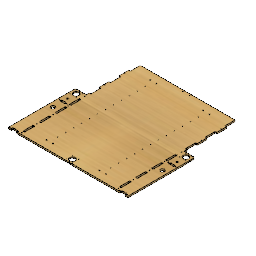
Bottom-plate-IIIS-rev1_8mm v1 (Autodesk Fusion 360 design; units mm, degrees)
Autodesk Fusion 360 part; units mm, degrees
(part 1 of 2)
sketch "Basic shape" plane through (0, 0, 0) normal (0, 1, 0) x (1, 0, 0)
  line L0 (-300, 300) -> (300, 300)
  line L1 (300, 300) -> (300, -300)
  line L2 (300, -300) -> (-300, -300)
  line L3 (-300, -300) -> (-300, 300)
  line L4 (-300, 300) -> (-246, 300)
  line L5 (-246, 300) -> (-246, 36.5)
  line L6 (-246, 36.5) -> (-300, 36.5)
  line L7 (-300, 36.5) -> (-300, 300)
  line L8 (300, 300) -> (246, 300)
  line L9 (246, 300) -> (246, 36.5)
  line L10 (246, 36.5) -> (300, 36.5)
  line L11 (300, 36.5) -> (300, 300)
  dimension "d1" = 600
  dimension "d2" = 600
  dimension "d3" = 263.5
  dimension "d4" = 54
  measures "d100" distance of origin
  measures "d166" distance of origin
extrude "Extrude1" add sketch "Basic shape" along normal blind 8 contours L0 L1 L2 L3 L5 L6 L9 L10
sketch "XZ1 plane projected" plane through (0, 8, 0) normal (0, 1, 0) x (-1, 0, 0)
  line L0 (246, -300) -> (246, -36.5)
  line L1 (246, -36.5) -> (300, -36.5)
  line L2 (300, -36.5) -> (300, 300)
  line L3 (300, 300) -> (-300, 300)
  line L4 (-300, 300) -> (-300, -36.5)
  line L5 (-300, -36.5) -> (-246, -36.5)
  line L6 (-246, -36.5) -> (-246, -300)
  line L7 (-246, -300) -> (246, -300)
  line L8 (300, 48.5) -> (-300, 48.5) construction
  line L9 (-300, 48.5) -> (-300, 56.5) construction
  line L10 (-300, 56.5) -> (300, 56.5) construction
  line L11 (300, 56.5) -> (300, 48.5) construction
  dimension "d29" = 48.5
  dimension "d30" = 8
sketch "XZ1 joints" plane through (0, 8, 0) normal (0, 1, 0) x (-1, 0, 0)
  line L0 (300, 48.5) -> (285.5, 48.5)
  line L1 (285.5, 48.5) -> (285.5, 56.5)
  line L2 (285.5, 56.5) -> (300, 56.5)
  line L3 (300, 56.5) -> (300, 48.5)
  line L4 (-300, 56.5) -> (300, 56.5)
  line L5 (260.5, 48.5) -> (246, 48.5)
  line L6 (246, 48.5) -> (246, 56.5)
  line L7 (246, 56.5) -> (260.5, 56.5)
  line L8 (260.5, 56.5) -> (260.5, 48.5)
  line L9 (300, 48.5) -> (-300, 48.5)
  dimension "d31" = 14.5
  dimension "d32" = 25
  dimension "d33" = 14.5
  measures "d32" distance of L1 L8
sketch "XZ1 joints holes" plane through (0, 8, 0) normal (0, 1, 0) x (-1, 0, 0)
  circle A0 centre (254.5, 52.5) radius 2
  circle A1 centre (291.5, 52.5) radius 2
  line L0 (246, -300) -> (246, -36.5)
  line L1 (246, -36.5) -> (300, -36.5)
  line L2 (300, -36.5) -> (300, 300)
  line L3 (300, 300) -> (-300, 300)
  line L4 (-300, 300) -> (-300, -36.5)
  line L5 (-300, -36.5) -> (-246, -36.5)
  line L6 (-246, -36.5) -> (-246, -300)
  line L7 (-246, -300) -> (246, -300)
  line L8 (300, 48.5) -> (285.5, 48.5)
  line L9 (260.5, 48.5) -> (246, 48.5)
  dimension "d34" = 4
  dimension "d64" = 4
  dimension "d71" = 4
  dimension "d72" = 4
  dimension "d1200" = 6
  dimension "d1201" = 6
  measures "d34" diameter of A0
  measures "d64" diameter of A1
extrude "Extrude2" cut sketch "XZ1 joints" sketch "XZ1 joints holes" against normal through all contours L1 L4 L8 L9 of sketch 2 contours A0 | A1
mirror "Mirror1" about plane through (0, 0, 0) normal (1, 0, 0) of "Extrude2"
sketch "XZ2 plane projected" plane through (0, 8, 0) normal (0, 1, 0) x (-1, 0, 0)
  line L0 (-246, -300) -> (246, -300)
  line L1 (246, -300) -> (246, -36.5)
  line L2 (246, -36.5) -> (300, -36.5)
  line L3 (300, -36.5) -> (300, 300)
  line L4 (300, 300) -> (-300, 300) construction
  line L5 (300, 300) -> (-300, 300) construction
  line L6 (-300, 300) -> (-300, 292) construction
  line L7 (-300, 292) -> (300, 292) construction
  line L8 (300, 292) -> (300, 300) construction
  dimension "d53" = 8
sketch "XZ2 joints" plane through (0, 8, 0) normal (0, 1, 0) x (-1, 0, 0)
  line L0 (-246, -300) -> (246, -300)
  line L1 (246, -300) -> (246, -36.5)
  line L2 (246, -36.5) -> (300, -36.5)
  line L3 (300, -36.5) -> (300, 300)
  line L4 (300, 300) -> (-300, 300)
  line L5 (300, 292) -> (285.5, 292)
  line L6 (285.5, 292) -> (285.5, 300)
  line L7 (285.5, 300) -> (300, 300)
  line L8 (300, 300) -> (300, 292)
  line L9 (260.5, 292) -> (246, 292)
  line L10 (246, 292) -> (246, 300)
  line L11 (246, 300) -> (260.5, 300)
  line L12 (260.5, 300) -> (260.5, 292)
  line L13 (-300, 292) -> (300, 292)
  dimension "d54" = 14.5
  dimension "d55" = 14.5
  dimension "d56" = 25
sketch "XZ2 joints holes" plane through (-273.5, 8, 295) normal (0, 1, 0) x (-1, 0, 0)
  circle A0 centre (18, 1) radius 2
  circle A1 centre (-19, 1) radius 2
  line L0 (26.5, -3) -> (12, -3)
  line L1 (-13, -3) -> (-27.5, -3)
  dimension "d73" = 4
  dimension "d74" = 4
  dimension "d75" = 4
  dimension "d76" = 4
  dimension "d77" = 6
  dimension "d78" = 6
  measures "d73" diameter of A0
  measures "d74" diameter of A1
  measures "d75" distance of L0
  measures "d76" distance of L1
extrude "Extrude3" cut sketch "XZ2 joints" sketch "XZ2 joints holes" against normal through all contours L4 L6 L12 L13 of sketch 2
mirror "Mirror2" about plane through (0, 0, 0) normal (1, 0, 0) of "Extrude3"
sketch "Square projected" plane through (0, 8, 0) normal (0, 1, 0) x (-1, 0, 0)
  circle A0 centre (291.5, 296) radius 2
  circle A1 centre (254.5, 296) radius 2
  circle A2 centre (-291.5, 52.5) radius 2
  line L0 (-260.5, 48.5) -> (-285.5, 48.5)
  line L1 (-285.5, 48.5) -> (-285.5, 56.5)
  line L2 (-285.5, 56.5) -> (-260.5, 56.5)
  line L3 (-260.5, 56.5) -> (-260.5, 48.5)
  circle A3 centre (-254.5, 52.5) radius 2
  circle A4 centre (291.5, 52.5) radius 2
  line L4 (260.5, 56.5) -> (285.5, 56.5)
  line L5 (285.5, 56.5) -> (285.5, 48.5)
  line L6 (285.5, 48.5) -> (260.5, 48.5)
  line L7 (260.5, 48.5) -> (260.5, 56.5)
  circle A5 centre (254.5, 52.5) radius 2
  line L8 (-260.5, 300) -> (-260.5, 292)
  line L9 (-260.5, 292) -> (-285.5, 292)
  line L10 (-285.5, 292) -> (-285.5, 300)
  line L11 (-285.5, 300) -> (-300, 300)
  line L12 (-300, 300) -> (-300, -36.5)
  line L13 (-300, -36.5) -> (-246, -36.5)
  line L14 (-246, -36.5) -> (-246, -300)
  line L15 (-246, -300) -> (246, -300)
  line L16 (246, -300) -> (246, -36.5)
  line L17 (246, -36.5) -> (300, -36.5)
  line L18 (300, -36.5) -> (300, 300)
  line L19 (300, 300) -> (285.5, 300)
  line L20 (285.5, 300) -> (285.5, 292)
  line L21 (285.5, 292) -> (260.5, 292)
  line L22 (260.5, 292) -> (260.5, 300)
  line L23 (260.5, 300) -> (-260.5, 300)
  circle A6 centre (-254.5, 296) radius 2
  circle A7 centre (-291.5, 296) radius 2
  line L24 (246, 300) -> (238, 300) construction
  line L25 (238, 300) -> (238, -300) construction
  line L26 (238, -300) -> (246, -300) construction
  line L27 (246, -300) -> (246, 300) construction
  dimension "d80" = 8
sketch "SquareBack joints" plane through (0, 8, 0) normal (0, 1, 0) x (-1, 0, 0)
  line L0 (246, 68.5) -> (238, 68.5)
  line L1 (238, 68.5) -> (238, 118.5)
  line L2 (238, 118.5) -> (246, 118.5)
  line L3 (246, 118.5) -> (246, 68.5)
  line L4 (246, -300) -> (246, 300)
  line L5 (238, 300) -> (238, -300)
  line L6 (246, 149.25) -> (238, 149.25)
  line L7 (238, 149.25) -> (238, 199.25)
  line L8 (238, 199.25) -> (246, 199.25)
  line L9 (246, 199.25) -> (246, 149.25)
  line L10 (246, 230) -> (238, 230)
  line L11 (238, 230) -> (238, 280)
  line L12 (238, 280) -> (246, 280)
  line L13 (246, 280) -> (246, 230)
  line L14 (238, 199.25) -> (238, 230) construction
  line L15 (238, 230) -> (238, 199.25)
  line L16 (238, 118.5) -> (238, 149.25) construction
  dimension "d81" = 50
  dimension "d1204" = 20
  dimension "d1205" = 20
  dimension "d1918" = 30.75
extrude "Extrude4" cut sketch "SquareBack joints" against normal through all contours L0 L1 L2 L3 L4 L5 | L4 L5 L6 L7 L8 L9 | L4 L5 L10 L11 L12 L13
sketch "SquareBack joints holes" plane through (0, 8, 0) normal (0, 1, 0) x (-1, 0, 0)
  line L0 (246, 68.5) -> (238, 68.5)
  line L1 (238, 68.5) -> (238, 118.5)
  line L2 (238, 118.5) -> (246, 118.5)
  line L3 (246, 118.5) -> (246, 68.5)
  line L4 (246, 199.25) -> (246, 149.25)
  line L5 (246, 149.25) -> (238, 149.25)
  line L6 (238, 149.25) -> (238, 199.25)
  line L7 (238, 199.25) -> (246, 199.25)
  line L8 (246, 280) -> (246, 230)
  line L9 (246, 230) -> (238, 230)
  line L10 (238, 230) -> (238, 280)
  line L11 (238, 280) -> (246, 280)
  circle A0 centre (291.5, 296) radius 2
  circle A1 centre (254.5, 296) radius 2
  circle A2 centre (-291.5, 52.5) radius 2
  line L12 (-260.5, 48.5) -> (-285.5, 48.5)
  line L13 (-285.5, 48.5) -> (-285.5, 56.5)
  line L14 (-285.5, 56.5) -> (-260.5, 56.5)
  line L15 (-260.5, 56.5) -> (-260.5, 48.5)
  circle A3 centre (-254.5, 52.5) radius 2
  circle A4 centre (291.5, 52.5) radius 2
  line L16 (260.5, 56.5) -> (285.5, 56.5)
  line L17 (285.5, 56.5) -> (285.5, 48.5)
  line L18 (285.5, 48.5) -> (260.5, 48.5)
  line L19 (260.5, 48.5) -> (260.5, 56.5)
  circle A5 centre (254.5, 52.5) radius 2
  line L20 (-260.5, 300) -> (-260.5, 292)
  line L21 (-260.5, 292) -> (-285.5, 292)
  line L22 (-285.5, 292) -> (-285.5, 300)
  line L23 (-285.5, 300) -> (-300, 300)
  line L24 (-300, 300) -> (-300, -36.5)
  line L25 (-300, -36.5) -> (-246, -36.5)
  line L26 (-246, -36.5) -> (-246, -300)
  line L27 (-246, -300) -> (246, -300)
  line L28 (246, -300) -> (246, -36.5)
  line L29 (246, -36.5) -> (300, -36.5)
  line L30 (300, -36.5) -> (300, 300)
  line L31 (300, 300) -> (285.5, 300)
  line L32 (285.5, 300) -> (285.5, 292)
  line L33 (285.5, 292) -> (260.5, 292)
  line L34 (260.5, 292) -> (260.5, 300)
  line L35 (260.5, 300) -> (-260.5, 300)
  circle A6 centre (-254.5, 296) radius 2
  circle A7 centre (-291.5, 296) radius 2
  circle A8 centre (242, 58.5) radius 2
  circle A9 centre (242, 133.875) radius 2
  circle A10 centre (242, 290) radius 2
  circle A11 centre (242, 214.625) radius 2
  line L36 (246, 68.5) -> (238, 68.5)
  line L37 (238, 118.5) -> (238, 149.25) construction
  line L38 (238, 199.25) -> (238, 230) construction
  dimension "d86" = 4
  dimension "d87" = 4
  dimension "d88" = 4
  dimension "d89" = 4
  dimension "d727" = 10
  dimension "d728" = 10
  dimension "d1206" = 14.625
  dimension "d1207" = 14.625
  dimension "d1208" = 14.625
  dimension "d1209" = 14.625
  measures "d86" diameter of A10
  measures "d87" diameter of A11
  measures "d88" diameter of A9
  measures "d89" diameter of A8
extrude "Extrude5" cut sketch "SquareBack joints holes" against normal through all contours A8 | A9 | A10 | A11
mirror "Mirror3" about plane through (0, 0, 0) normal (1, 0, 0) of "Extrude4", "Extrude5"
sketch "SquareFront joints" plane through (0, 0, 0) normal (0, 1, 0) x (1, 0, 0)
  line L0 (-238, 300) -> (-246, 300)
  line L1 (-246, 300) -> (-246, 200.5)
  line L2 (-246, 200.5) -> (-238, 200.5)
  line L3 (-238, 200.5) -> (-238, 300)
  line L4 (-246, 300) -> (-246, 36.5)
  line L5 (-246, 300) -> (-246, -300)
  line L6 (-238, 250) -> (-246, 250)
  line L7 (-246, 250) -> (-246, 150.5)
  line L8 (-246, 150.5) -> (-238, 150.5)
  line L9 (-238, 150.5) -> (-238, 250)
  line L10 (-238, -300) -> (-238, 300)
  line L11 (-238, 101) -> (-246, 101)
  line L12 (-246, 101) -> (-246, 51)
  line L13 (-246, 51) -> (-238, 51)
  line L14 (-238, 51) -> (-238, 101)
  line L15 (-238, 1.5) -> (-246, 1.5)
  line L16 (-246, 1.5) -> (-246, -48.5)
  line L17 (-246, -48.5) -> (-238, -48.5)
  line L18 (-238, -48.5) -> (-238, 1.5)
  line L19 (-238, 200.5) -> (-238, 250) construction
  line L20 (-238, 150.5) -> (-238, 101) construction
  line L21 (-238, 51) -> (-238, 1.5) construction
  dimension "d94" = 50
  dimension "d98" = 50
  dimension "d99" = 50
  dimension "d100" = 50
  measures "d98" distance of L2 L8
  measures "d99" distance of L11 L13
  measures "d100" distance of L15 L17
extrude "Extrude6" cut sketch "SquareFront joints" along normal through all contours L0 L1 L3 L4 L5 L6 L10 | L2 L4 L5 L7 L8 L9 L10 | L4 L5 L10 L11 L12 L13 L14 | L5 L10 L15 L16 L17 L18
sketch "SquareFront joints holes" plane through (0, 0, 0) normal (0, -1, 0) x (1, 0, 0)
  circle A0 centre (-254.5, 52.5) radius 2
  line L0 (-285.5, 56.5) -> (-260.5, 56.5)
  line L1 (-260.5, 56.5) -> (-260.5, 48.5)
  line L2 (-260.5, 48.5) -> (-285.5, 48.5)
  line L3 (-285.5, 48.5) -> (-285.5, 56.5)
  circle A1 centre (-291.5, 52.5) radius 2
  circle A2 centre (254.5, 52.5) radius 2
  line L4 (285.5, 48.5) -> (260.5, 48.5)
  line L5 (260.5, 48.5) -> (260.5, 56.5)
  line L6 (260.5, 56.5) -> (285.5, 56.5)
  line L7 (285.5, 56.5) -> (285.5, 48.5)
  circle A3 centre (291.5, 52.5) radius 2
  circle A4 centre (-254.5, 296) radius 2
  circle A5 centre (-291.5, 296) radius 2
  circle A6 centre (254.5, 296) radius 2
  circle A7 centre (291.5, 296) radius 2
  line L8 (-246, 230) -> (-246, 280)
  line L9 (-246, 280) -> (-238, 280)
  line L10 (-238, 280) -> (-238, 230)
  line L11 (-238, 230) -> (-246, 230)
  line L12 (-246, 149.25) -> (-246, 199.25)
  line L13 (-246, 199.25) -> (-238, 199.25)
  line L14 (-238, 199.25) -> (-238, 149.25)
  line L15 (-238, 149.25) -> (-246, 149.25)
  line L16 (-238, 68.5) -> (-246, 68.5)
  line L17 (-246, 68.5) -> (-246, 118.5)
  line L18 (-246, 118.5) -> (-238, 118.5)
  line L19 (-238, 118.5) -> (-238, 68.5)
  circle A8 centre (-242, 290) radius 2
  circle A9 centre (-242, 58.5) radius 2
  circle A10 centre (-242, 214.625) radius 2
  circle A11 centre (-242, 133.875) radius 2
  line L20 (238, 230) -> (238, 280)
  line L21 (238, 280) -> (246, 280)
  line L22 (246, 280) -> (246, 230)
  line L23 (246, 230) -> (238, 230)
  line L24 (238, 149.25) -> (238, 199.25)
  line L25 (238, 199.25) -> (246, 199.25)
  line L26 (246, 199.25) -> (246, 149.25)
  line L27 (246, 149.25) -> (238, 149.25)
  line L28 (238, 118.5) -> (246, 118.5)
  line L29 (246, 118.5) -> (246, 68.5)
  line L30 (246, 68.5) -> (238, 68.5)
  line L31 (238, 68.5) -> (238, 118.5)
  circle A12 centre (242, 290) radius 2
  circle A13 centre (242, 58.5) radius 2
  circle A14 centre (242, 214.625) radius 2
  circle A15 centre (242, 133.875) radius 2
  line L32 (-246, 48.5) -> (-238, 48.5)
  line L33 (-238, 48.5) -> (-238, -1.5)
  line L34 (-238, -1.5) -> (-246, -1.5)
  line L35 (-246, -1.5) -> (-246, 48.5)
  line L36 (246, -300) -> (246, -36.5)
  line L37 (246, -36.5) -> (300, -36.5)
  line L38 (300, -36.5) -> (300, 300)
  line L39 (300, 300) -> (285.5, 300)
  line L40 (285.5, 300) -> (285.5, 292)
  line L41 (285.5, 292) -> (260.5, 292)
  line L42 (260.5, 292) -> (260.5, 300)
  line L43 (260.5, 300) -> (-260.5, 300)
  line L44 (-260.5, 300) -> (-260.5, 292)
  line L45 (-260.5, 292) -> (-285.5, 292)
  line L46 (-285.5, 292) -> (-285.5, 300)
  line L47 (-285.5, 300) -> (-300, 300)
  line L48 (-300, 300) -> (-300, -36.5)
  line L49 (-300, -36.5) -> (-246, -36.5)
  line L50 (-246, -36.5) -> (-246, -51)
  line L51 (-246, -51) -> (-238, -51)
  line L52 (-238, -51) -> (-238, -101)
  line L53 (-238, -101) -> (-246, -101)
  line L54 (-246, -101) -> (-246, -150.5)
  line L55 (-246, -150.5) -> (-238, -150.5)
  line L56 (-238, -150.5) -> (-238, -200.5)
  line L57 (-238, -200.5) -> (-246, -200.5)
  line L58 (-246, -200.5) -> (-246, -250)
  line L59 (-246, -250) -> (-238, -250)
  line L60 (-238, -250) -> (-238, -300)
  line L61 (-238, -300) -> (246, -300)
  circle A16 centre (-242, -225.25) radius 2
  circle A17 centre (-242, -125.75) radius 2
  circle A18 centre (-242, -26.25) radius 2
  line L62 (-238, -250) -> (-238, -200.5) construction
  line L63 (-238, -150.5) -> (-238, -101) construction
  line L64 (-238, -51) -> (-238, -1.5) construction
  dimension "d105" = 4
  dimension "d106" = 4
  dimension "d107" = 4
  dimension "d108" = 4
  dimension "d109" = 4
  dimension "d110" = 4
  measures "d108" diameter of A18
  measures "d109" diameter of A17
  measures "d110" diameter of A16
extrude "Extrude7" cut sketch "SquareFront joints holes" against normal through all contours A16 | A17 | A18
mirror "Mirror5" about plane through (0, 0, 0) normal (1, 0, 0) of "Extrude6", "Extrude7"
sketch "SK8" plane through (0, 8, 0) normal (0, 1, 0) x (-1, 0, 0)
  circle A0 centre (-242, -225.25) radius 2
  circle A1 centre (-242, -125.75) radius 2
  circle A2 centre (-242, -26.25) radius 2
  circle A3 centre (242, -225.25) radius 2
  circle A4 centre (242, -125.75) radius 2
  circle A5 centre (242, -26.25) radius 2
  circle A6 centre (-242, 133.875) radius 2
  circle A7 centre (-242, 214.625) radius 2
  circle A8 centre (-242, 58.5) radius 2
  circle A9 centre (-242, 290) radius 2
  line L0 (-246, 118.5) -> (-238, 118.5)
  line L1 (-238, 118.5) -> (-238, 68.5)
  line L2 (-238, 68.5) -> (-246, 68.5)
  line L3 (-246, 68.5) -> (-246, 118.5)
  line L4 (-238, 199.25) -> (-238, 149.25)
  line L5 (-238, 149.25) -> (-246, 149.25)
  line L6 (-246, 149.25) -> (-246, 199.25)
  line L7 (-246, 199.25) -> (-238, 199.25)
  line L8 (-238, 280) -> (-238, 230)
  line L9 (-238, 230) -> (-246, 230)
  line L10 (-246, 230) -> (-246, 280)
  line L11 (-246, 280) -> (-238, 280)
  circle A10 centre (242, 133.875) radius 2
  circle A11 centre (242, 214.625) radius 2
  circle A12 centre (242, 58.5) radius 2
  circle A13 centre (242, 290) radius 2
  line L12 (246, 68.5) -> (238, 68.5)
  line L13 (238, 68.5) -> (238, 118.5)
  line L14 (238, 118.5) -> (246, 118.5)
  line L15 (246, 118.5) -> (246, 68.5)
  line L16 (246, 199.25) -> (246, 149.25)
  line L17 (246, 149.25) -> (238, 149.25)
  line L18 (238, 149.25) -> (238, 199.25)
  line L19 (238, 199.25) -> (246, 199.25)
  line L20 (246, 280) -> (246, 230)
  line L21 (246, 230) -> (238, 230)
  line L22 (238, 230) -> (238, 280)
  line L23 (238, 280) -> (246, 280)
  circle A14 centre (291.5, 296) radius 2
  circle A15 centre (254.5, 296) radius 2
  circle A16 centre (-291.5, 52.5) radius 2
  line L24 (-260.5, 48.5) -> (-285.5, 48.5)
  line L25 (-285.5, 48.5) -> (-285.5, 56.5)
  line L26 (-285.5, 56.5) -> (-260.5, 56.5)
  line L27 (-260.5, 56.5) -> (-260.5, 48.5)
  circle A17 centre (-254.5, 52.5) radius 2
  circle A18 centre (291.5, 52.5) radius 2
  line L28 (260.5, 56.5) -> (285.5, 56.5)
  line L29 (285.5, 56.5) -> (285.5, 48.5)
  line L30 (285.5, 48.5) -> (260.5, 48.5)
  line L31 (260.5, 48.5) -> (260.5, 56.5)
  circle A19 centre (254.5, 52.5) radius 2
  line L32 (-260.5, 300) -> (-260.5, 292)
  line L33 (-260.5, 292) -> (-285.5, 292)
  line L34 (-285.5, 292) -> (-285.5, 300)
  line L35 (-285.5, 300) -> (-300, 300)
  line L36 (-300, 300) -> (-300, -36.5)
  line L37 (-300, -36.5) -> (-246, -36.5)
  line L38 (-246, -36.5) -> (-246, -51)
  line L39 (-238, -300) -> (238, -300)
  line L40 (246, -250) -> (246, -200.5)
  line L41 (246, -36.5) -> (300, -36.5)
  line L42 (300, -36.5) -> (300, 300)
  line L43 (300, 300) -> (285.5, 300)
  line L44 (285.5, 300) -> (285.5, 292)
  line L45 (285.5, 292) -> (260.5, 292)
  line L46 (260.5, 292) -> (260.5, 300)
  line L47 (260.5, 300) -> (-260.5, 300)
  circle A20 centre (-254.5, 296) radius 2
  circle A21 centre (-291.5, 296) radius 2
  line L48 (-149, -260) -> (-117, -260) construction
  circle A22 centre (-149, -260) radius 2.5
  circle A23 centre (-117, -260) radius 2.5
  line L49 (246, -1.5) -> (238, -1.5)
  line L50 (238, -1.5) -> (238, 48.5)
  line L51 (238, 48.5) -> (246, 48.5)
  line L52 (246, 48.5) -> (246, -1.5)
  line L53 (-246, 48.5) -> (-238, 48.5)
  line L54 (-238, 48.5) -> (-238, -1.5)
  line L55 (-238, -1.5) -> (-246, -1.5)
  line L56 (-246, -1.5) -> (-246, 48.5)
  line L57 (-246, -250) -> (-238, -250)
  line L58 (-238, -250) -> (-238, -300)
  line L59 (238, -300) -> (238, -250)
  line L60 (238, -250) -> (246, -250)
  line L61 (246, -200.5) -> (238, -200.5)
  line L62 (238, -200.5) -> (238, -150.5)
  line L63 (238, -150.5) -> (246, -150.5)
  line L64 (246, -150.5) -> (246, -101)
  line L65 (246, -101) -> (238, -101)
  line L66 (238, -101) -> (238, -51)
  line L67 (238, -51) -> (246, -51)
  line L68 (246, -51) -> (246, -36.5)
  line L69 (-246, -51) -> (-238, -51)
  line L70 (-238, -51) -> (-238, -101)
  line L71 (-238, -101) -> (-246, -101)
  line L72 (-246, -101) -> (-246, -150.5)
  line L73 (-246, -150.5) -> (-238, -150.5)
  line L74 (-238, -150.5) -> (-238, -200.5)
  line L75 (-238, -200.5) -> (-246, -200.5)
  line L76 (-246, -200.5) -> (-246, -250)
  dimension "d113" = 5
  dimension "d114" = 5
  dimension "d115" = 32
  dimension "d116" = 40
  dimension "d117" = 133
  dimension "d130" = 200
  measures "d113" diameter of A22
  measures "d114" diameter of A23
  measures "d116" distance of L39 L48
extrude "Extrude8" cut sketch "SK8" against normal through all contours A22 | A23
mirror "Mirror6" about plane through (0, 0, 0) normal (1, 0, 0) of "Extrude8"
mirror "Mirror7" about plane through (0, 0, 0) normal (0, 0, 1) of "Extrude8"
mirror "Mirror8" about plane through (0, 0, 0) normal (0, 0, 1) of "Mirror6"
sketch "Linear rail" plane through (0, 8, 0) normal (0, 1, 0) x (-1, 0, 0)
  circle A0 centre (149, 260) radius 2.5
  circle A1 centre (117, 260) radius 2.5
  circle A2 centre (-149, 260) radius 2.5
  circle A3 centre (-117, 260) radius 2.5
  circle A4 centre (149, -260) radius 2.5
  circle A5 centre (117, -260) radius 2.5
  circle A6 centre (-149, -260) radius 2.5
  circle A7 centre (-117, -260) radius 2.5
  circle A8 centre (-242, -225.25) radius 2
  circle A9 centre (-242, -125.75) radius 2
  circle A10 centre (-242, -26.25) radius 2
  circle A11 centre (242, -225.25) radius 2
  circle A12 centre (242, -125.75) radius 2
  circle A13 centre (242, -26.25) radius 2
  circle A14 centre (-242, 133.875) radius 2
  circle A15 centre (-242, 214.625) radius 2
  circle A16 centre (-242, 58.5) radius 2
  circle A17 centre (-242, 290) radius 2
  line L0 (-246, 118.5) -> (-238, 118.5)
  line L1 (-238, 118.5) -> (-238, 68.5)
  line L2 (-238, 68.5) -> (-246, 68.5)
  line L3 (-246, 68.5) -> (-246, 118.5)
  line L4 (-238, 199.25) -> (-238, 149.25)
  line L5 (-238, 149.25) -> (-246, 149.25)
  line L6 (-246, 149.25) -> (-246, 199.25)
  line L7 (-246, 199.25) -> (-238, 199.25)
  line L8 (-238, 280) -> (-238, 230)
  line L9 (-238, 230) -> (-246, 230)
  line L10 (-246, 230) -> (-246, 280)
  line L11 (-246, 280) -> (-238, 280)
  circle A18 centre (242, 133.875) radius 2
  circle A19 centre (242, 214.625) radius 2
  circle A20 centre (242, 58.5) radius 2
  circle A21 centre (242, 290) radius 2
  line L12 (246, 68.5) -> (238, 68.5)
  line L13 (238, 68.5) -> (238, 118.5)
  line L14 (238, 118.5) -> (246, 118.5)
  line L15 (246, 118.5) -> (246, 68.5)
  line L16 (246, 199.25) -> (246, 149.25)
  line L17 (246, 149.25) -> (238, 149.25)
  line L18 (238, 149.25) -> (238, 199.25)
  line L19 (238, 199.25) -> (246, 199.25)
  line L20 (246, 280) -> (246, 230)
  line L21 (246, 230) -> (238, 230)
  line L22 (238, 230) -> (238, 280)
  line L23 (238, 280) -> (246, 280)
  circle A22 centre (291.5, 296) radius 2
  circle A23 centre (254.5, 296) radius 2
  circle A24 centre (-291.5, 52.5) radius 2
  line L24 (-260.5, 48.5) -> (-285.5, 48.5)
  line L25 (-285.5, 48.5) -> (-285.5, 56.5)
  line L26 (-285.5, 56.5) -> (-260.5, 56.5)
  line L27 (-260.5, 56.5) -> (-260.5, 48.5)
  circle A25 centre (-254.5, 52.5) radius 2
  circle A26 centre (291.5, 52.5) radius 2
  line L28 (260.5, 56.5) -> (285.5, 56.5)
  line L29 (285.5, 56.5) -> (285.5, 48.5)
  line L30 (285.5, 48.5) -> (260.5, 48.5)
  line L31 (260.5, 48.5) -> (260.5, 56.5)
  circle A27 centre (254.5, 52.5) radius 2
  line L32 (-260.5, 300) -> (-260.5, 292)
  line L33 (-260.5, 292) -> (-285.5, 292)
  line L34 (-285.5, 292) -> (-285.5, 300)
  line L35 (-285.5, 300) -> (-300, 300)
  line L36 (-300, 300) -> (-300, -36.5)
  line L37 (-300, -36.5) -> (-246, -36.5)
  line L38 (-246, -36.5) -> (-246, -51)
  line L39 (-238, -300) -> (238, -300)
  line L40 (246, -250) -> (246, -200.5)
  line L41 (246, -36.5) -> (300, -36.5)
  line L42 (300, -36.5) -> (300, 300)
  line L43 (300, 300) -> (285.5, 300)
  line L44 (285.5, 300) -> (285.5, 292)
  line L45 (285.5, 292) -> (260.5, 292)
  line L46 (260.5, 292) -> (260.5, 300)
  line L47 (260.5, 300) -> (-260.5, 300)
  circle A28 centre (-254.5, 296) radius 2
  circle A29 centre (-291.5, 296) radius 2
  circle A30 centre (-133, -220) radius 1.5
  line L48 (246, -1.5) -> (238, -1.5)
  line L49 (238, -1.5) -> (238, 48.5)
  line L50 (238, 48.5) -> (246, 48.5)
  line L51 (246, 48.5) -> (246, -1.5)
  line L52 (-246, 48.5) -> (-238, 48.5)
  line L53 (-238, 48.5) -> (-238, -1.5)
  line L54 (-238, -1.5) -> (-246, -1.5)
  line L55 (-246, -1.5) -> (-246, 48.5)
  line L56 (-246, -250) -> (-238, -250)
  line L57 (-238, -250) -> (-238, -300)
  line L58 (238, -300) -> (238, -250)
  line L59 (238, -250) -> (246, -250)
  line L60 (246, -200.5) -> (238, -200.5)
  line L61 (238, -200.5) -> (238, -150.5)
  line L62 (238, -150.5) -> (246, -150.5)
  line L63 (246, -150.5) -> (246, -101)
  line L64 (246, -101) -> (238, -101)
  line L65 (238, -101) -> (238, -51)
  line L66 (238, -51) -> (246, -51)
  line L67 (246, -51) -> (246, -36.5)
  line L68 (-246, -51) -> (-238, -51)
  line L69 (-238, -51) -> (-238, -101)
  line L70 (-238, -101) -> (-246, -101)
  line L71 (-246, -101) -> (-246, -150.5)
  line L72 (-246, -150.5) -> (-238, -150.5)
  line L73 (-238, -150.5) -> (-238, -200.5)
  line L74 (-238, -200.5) -> (-246, -200.5)
  line L75 (-246, -200.5) -> (-246, -250)
  dimension "d123" = 133
  dimension "d124" = 3
  dimension "d131" = 80
  measures "d124" diameter of A30
extrude "Extrude9" cut sketch "Linear rail" against normal through all contours A30
pattern_linear "R-Pattern1" count 12 spacing 40 along (0, 0, 1) of "Extrude9"
mirror "Mirror9" about plane through (0, 0, 0) normal (1, 0, 0) of "Extrude9", "R-Pattern1"
sketch "Y cable stretcher" plane through (0, 8, 0) normal (0, 1, 0) x (-1, 0, 0)
  circle A0 centre (133, 100) radius 1.5
  circle A1 centre (133, 60) radius 1.5
  circle A2 centre (133, 20) radius 1.5
  circle A3 centre (133, -20) radius 1.5
  circle A4 centre (133, -60) radius 1.5
  circle A5 centre (133, -100) radius 1.5
  circle A6 centre (133, -140) radius 1.5
  circle A7 centre (133, -180) radius 1.5
  circle A8 centre (133, -220) radius 1.5
  circle A9 centre (-133, 100) radius 1.5
  circle A10 centre (-133, 60) radius 1.5
  circle A11 centre (-133, 20) radius 1.5
  circle A12 centre (-133, -20) radius 1.5
  circle A13 centre (-133, -60) radius 1.5
  circle A14 centre (-133, -100) radius 1.5
  circle A15 centre (-133, -140) radius 1.5
  circle A16 centre (-133, -180) radius 1.5
  circle A17 centre (-133, -220) radius 1.5
  circle A18 centre (149, 260) radius 2.5
  circle A19 centre (117, 260) radius 2.5
  circle A20 centre (-149, 260) radius 2.5
  circle A21 centre (-117, 260) radius 2.5
  circle A22 centre (149, -260) radius 2.5
  circle A23 centre (117, -260) radius 2.5
  circle A24 centre (-149, -260) radius 2.5
  circle A25 centre (-117, -260) radius 2.5
  circle A26 centre (-242, -225.25) radius 2
  circle A27 centre (-242, -125.75) radius 2
  circle A28 centre (-242, -26.25) radius 2
  circle A29 centre (242, -225.25) radius 2
  circle A30 centre (242, -125.75) radius 2
  circle A31 centre (242, -26.25) radius 2
  circle A32 centre (-242, 133.875) radius 2
  circle A33 centre (-242, 214.625) radius 2
  circle A34 centre (-242, 58.5) radius 2
  circle A35 centre (-242, 290) radius 2
  line L0 (-246, 118.5) -> (-238, 118.5)
  line L1 (-238, 118.5) -> (-238, 68.5)
  line L2 (-238, 68.5) -> (-246, 68.5)
  line L3 (-246, 68.5) -> (-246, 118.5)
  line L4 (-238, 199.25) -> (-238, 149.25)
  line L5 (-238, 149.25) -> (-246, 149.25)
  line L6 (-246, 149.25) -> (-246, 199.25)
  line L7 (-246, 199.25) -> (-238, 199.25)
  line L8 (-238, 280) -> (-238, 230)
  line L9 (-238, 230) -> (-246, 230)
  line L10 (-246, 230) -> (-246, 280)
  line L11 (-246, 280) -> (-238, 280)
  circle A36 centre (242, 133.875) radius 2
  circle A37 centre (242, 214.625) radius 2
  circle A38 centre (242, 58.5) radius 2
  circle A39 centre (242, 290) radius 2
  line L12 (246, 68.5) -> (238, 68.5)
  line L13 (238, 68.5) -> (238, 118.5)
  line L14 (238, 118.5) -> (246, 118.5)
  line L15 (246, 118.5) -> (246, 68.5)
  line L16 (246, 199.25) -> (246, 149.25)
  line L17 (246, 149.25) -> (238, 149.25)
  line L18 (238, 149.25) -> (238, 199.25)
  line L19 (238, 199.25) -> (246, 199.25)
  line L20 (246, 280) -> (246, 230)
  line L21 (246, 230) -> (238, 230)
  line L22 (238, 230) -> (238, 280)
  line L23 (238, 280) -> (246, 280)
  circle A40 centre (291.5, 296) radius 2
  circle A41 centre (254.5, 296) radius 2
  circle A42 centre (-291.5, 52.5) radius 2
  line L24 (-260.5, 48.5) -> (-285.5, 48.5)
  line L25 (-285.5, 48.5) -> (-285.5, 56.5)
  line L26 (-285.5, 56.5) -> (-260.5, 56.5)
  line L27 (-260.5, 56.5) -> (-260.5, 48.5)
  circle A43 centre (-254.5, 52.5) radius 2
  circle A44 centre (291.5, 52.5) radius 2
  line L28 (260.5, 56.5) -> (285.5, 56.5)
  line L29 (285.5, 56.5) -> (285.5, 48.5)
  line L30 (285.5, 48.5) -> (260.5, 48.5)
  line L31 (260.5, 48.5) -> (260.5, 56.5)
  circle A45 centre (254.5, 52.5) radius 2
  line L32 (-260.5, 300) -> (-260.5, 292)
  line L33 (-260.5, 292) -> (-285.5, 292)
  line L34 (-285.5, 292) -> (-285.5, 300)
  line L35 (-285.5, 300) -> (-300, 300)
  line L36 (-300, 300) -> (-300, -36.5)
  line L37 (-300, -36.5) -> (-246, -36.5)
  line L38 (-246, -36.5) -> (-246, -51)
  line L39 (-238, -300) -> (238, -300)
  line L40 (246, -250) -> (246, -200.5)
  line L41 (246, -36.5) -> (300, -36.5)
  line L42 (300, -36.5) -> (300, 300)
  line L43 (300, 300) -> (285.5, 300)
  line L44 (285.5, 300) -> (285.5, 292)
  line L45 (285.5, 292) -> (260.5, 292)
  line L46 (260.5, 292) -> (260.5, 300)
  line L47 (260.5, 300) -> (-260.5, 300)
  circle A46 centre (-254.5, 296) radius 2
  circle A47 centre (-291.5, 296) radius 2
  circle A48 centre (133, 140) radius 1.5
  circle A49 centre (-133, 140) radius 1.5
  circle A50 centre (133, 180) radius 1.5
  circle A51 centre (-133, 180) radius 1.5
  circle A52 centre (-16, -292.5) radius 2
  circle A53 centre (133, 220) radius 1.5
  circle A54 centre (-133, 220) radius 1.5
  line L48 (246, -1.5) -> (238, -1.5)
  line L49 (238, -1.5) -> (238, 48.5)
  line L50 (238, 48.5) -> (246, 48.5)
  line L51 (246, 48.5) -> (246, -1.5)
  line L52 (-246, 48.5) -> (-238, 48.5)
  line L53 (-238, 48.5) -> (-238, -1.5)
  line L54 (-238, -1.5) -> (-246, -1.5)
  line L55 (-246, -1.5) -> (-246, 48.5)
  line L56 (-246, -250) -> (-238, -250)
  line L57 (-238, -250) -> (-238, -300)
  line L58 (238, -300) -> (238, -250)
  line L59 (238, -250) -> (246, -250)
  line L60 (246, -200.5) -> (238, -200.5)
  line L61 (238, -200.5) -> (238, -150.5)
  line L62 (238, -150.5) -> (246, -150.5)
  line L63 (246, -150.5) -> (246, -101)
  line L64 (246, -101) -> (238, -101)
  line L65 (238, -101) -> (238, -51)
  line L66 (238, -51) -> (246, -51)
  line L67 (246, -51) -> (246, -36.5)
  line L68 (-246, -51) -> (-238, -51)
  line L69 (-238, -51) -> (-238, -101)
  line L70 (-238, -101) -> (-246, -101)
  line L71 (-246, -101) -> (-246, -150.5)
  line L72 (-246, -150.5) -> (-238, -150.5)
  line L73 (-238, -150.5) -> (-238, -200.5)
  line L74 (-238, -200.5) -> (-246, -200.5)
  line L75 (-246, -200.5) -> (-246, -250)
  dimension "d134" = 7.5
  dimension "d732" = 4
  dimension "d733" = 16
  measures "d732" diameter of A52
  measures "d733" distance of origin
extrude "Extrude10" cut sketch "Y cable stretcher" against normal through all contours A52
mirror "Mirror10" about plane through (0, 0, 0) normal (1, 0, 0) of "Extrude10"
sketch "To pass cables" plane through (0, 8, 0) normal (0, 1, 0) x (-1, 0, 0)
  circle A0 centre (133, 100) radius 1.5
  circle A1 centre (133, 60) radius 1.5
  circle A2 centre (133, 20) radius 1.5
  circle A3 centre (133, -20) radius 1.5
  circle A4 centre (133, -60) radius 1.5
  circle A5 centre (133, -100) radius 1.5
  circle A6 centre (133, -140) radius 1.5
  circle A7 centre (133, -180) radius 1.5
  circle A8 centre (133, -220) radius 1.5
  circle A9 centre (-133, 100) radius 1.5
  circle A10 centre (-133, 60) radius 1.5
  circle A11 centre (-133, 20) radius 1.5
  circle A12 centre (-133, -20) radius 1.5
  circle A13 centre (-133, -60) radius 1.5
  circle A14 centre (-133, -100) radius 1.5
  circle A15 centre (-133, -140) radius 1.5
  circle A16 centre (-133, -180) radius 1.5
  circle A17 centre (-133, -220) radius 1.5
  circle A18 centre (149, 260) radius 2.5
  circle A19 centre (117, 260) radius 2.5
  circle A20 centre (-149, 260) radius 2.5
  circle A21 centre (-117, 260) radius 2.5
  circle A22 centre (149, -260) radius 2.5
  circle A23 centre (117, -260) radius 2.5
  circle A24 centre (-149, -260) radius 2.5
  circle A25 centre (-117, -260) radius 2.5
  circle A26 centre (-242, -225.25) radius 2
  circle A27 centre (-242, -125.75) radius 2
  circle A28 centre (-242, -26.25) radius 2
  circle A29 centre (242, -225.25) radius 2
  circle A30 centre (242, -125.75) radius 2
  circle A31 centre (242, -26.25) radius 2
  circle A32 centre (-242, 133.875) radius 2
  circle A33 centre (-242, 214.625) radius 2
  circle A34 centre (-242, 58.5) radius 2
  circle A35 centre (-242, 290) radius 2
  line L0 (-246, 118.5) -> (-238, 118.5)
  line L1 (-238, 118.5) -> (-238, 68.5)
  line L2 (-238, 68.5) -> (-246, 68.5)
  line L3 (-246, 68.5) -> (-246, 118.5)
  line L4 (-238, 199.25) -> (-238, 149.25)
  line L5 (-238, 149.25) -> (-246, 149.25)
  line L6 (-246, 149.25) -> (-246, 199.25)
  line L7 (-246, 199.25) -> (-238, 199.25)
  line L8 (-238, 280) -> (-238, 230)
  line L9 (-238, 230) -> (-246, 230)
  line L10 (-246, 230) -> (-246, 280)
  line L11 (-246, 280) -> (-238, 280)
  circle A36 centre (242, 133.875) radius 2
  circle A37 centre (242, 214.625) radius 2
  circle A38 centre (242, 58.5) radius 2
  circle A39 centre (242, 290) radius 2
  line L12 (246, 68.5) -> (238, 68.5)
  line L13 (238, 68.5) -> (238, 118.5)
  line L14 (238, 118.5) -> (246, 118.5)
  line L15 (246, 118.5) -> (246, 68.5)
  line L16 (246, 199.25) -> (246, 149.25)
  line L17 (246, 149.25) -> (238, 149.25)
  line L18 (238, 149.25) -> (238, 199.25)
  line L19 (238, 199.25) -> (246, 199.25)
  line L20 (246, 280) -> (246, 230)
  line L21 (246, 230) -> (238, 230)
  line L22 (238, 230) -> (238, 280)
  line L23 (238, 280) -> (246, 280)
  circle A40 centre (291.5, 296) radius 2
  circle A41 centre (254.5, 296) radius 2
  circle A42 centre (-291.5, 52.5) radius 2
  line L24 (-260.5, 48.5) -> (-285.5, 48.5)
  line L25 (-285.5, 48.5) -> (-285.5, 56.5)
  line L26 (-285.5, 56.5) -> (-260.5, 56.5)
  line L27 (-260.5, 56.5) -> (-260.5, 48.5)
  circle A43 centre (-254.5, 52.5) radius 2
  circle A44 centre (291.5, 52.5) radius 2
  line L28 (260.5, 56.5) -> (285.5, 56.5)
  line L29 (285.5, 56.5) -> (285.5, 48.5)
  line L30 (285.5, 48.5) -> (260.5, 48.5)
  line L31 (260.5, 48.5) -> (260.5, 56.5)
  circle A45 centre (254.5, 52.5) radius 2
  line L32 (-260.5, 300) -> (-260.5, 292)
  line L33 (-260.5, 292) -> (-285.5, 292)
  line L34 (-285.5, 292) -> (-285.5, 300)
  line L35 (-285.5, 300) -> (-300, 300)
  line L36 (-300, 300) -> (-300, -36.5)
  line L37 (-300, -36.5) -> (-246, -36.5)
  line L38 (-246, -36.5) -> (-246, -51)
  line L39 (-238, -300) -> (238, -300)
  line L40 (246, -250) -> (246, -200.5)
  line L41 (246, -36.5) -> (300, -36.5)
  line L42 (300, -36.5) -> (300, 300)
  line L43 (300, 300) -> (285.5, 300)
  line L44 (285.5, 300) -> (285.5, 292)
  line L45 (285.5, 292) -> (260.5, 292)
  line L46 (260.5, 292) -> (260.5, 300)
  line L47 (260.5, 300) -> (-260.5, 300)
  circle A46 centre (-254.5, 296) radius 2
  circle A47 centre (-291.5, 296) radius 2
  circle A48 centre (-275, 101.5) radius 10
  circle A49 centre (133, 140) radius 1.5
  circle A50 centre (-133, 140) radius 1.5
  circle A51 centre (133, 180) radius 1.5
  circle A52 centre (-133, 180) radius 1.5
  circle A53 centre (16, -292.5) radius 2
  circle A54 centre (-16, -292.5) radius 2
  circle A55 centre (133, 220) radius 1.5
  circle A56 centre (-133, 220) radius 1.5
  line L48 (246, -1.5) -> (238, -1.5)
  line L49 (238, -1.5) -> (238, 48.5)
  line L50 (238, 48.5) -> (246, 48.5)
  line L51 (246, 48.5) -> (246, -1.5)
  line L52 (-246, 48.5) -> (-238, 48.5)
  line L53 (-238, 48.5) -> (-238, -1.5)
  line L54 (-238, -1.5) -> (-246, -1.5)
  line L55 (-246, -1.5) -> (-246, 48.5)
  line L56 (-246, -250) -> (-238, -250)
  line L57 (-238, -250) -> (-238, -300)
  line L58 (238, -300) -> (238, -250)
  line L59 (238, -250) -> (246, -250)
  line L60 (246, -200.5) -> (238, -200.5)
  line L61 (238, -200.5) -> (238, -150.5)
  line L62 (238, -150.5) -> (246, -150.5)
  line L63 (246, -150.5) -> (246, -101)
  line L64 (246, -101) -> (238, -101)
  line L65 (238, -101) -> (238, -51)
  line L66 (238, -51) -> (246, -51)
  line L67 (246, -51) -> (246, -36.5)
  line L68 (-246, -51) -> (-238, -51)
  line L69 (-238, -51) -> (-238, -101)
  line L70 (-238, -101) -> (-246, -101)
  line L71 (-246, -101) -> (-246, -150.5)
  line L72 (-246, -150.5) -> (-238, -150.5)
  line L73 (-238, -150.5) -> (-238, -200.5)
  line L74 (-238, -200.5) -> (-246, -200.5)
  line L75 (-246, -200.5) -> (-246, -250)
  dimension "d139" = 20
  dimension "d140" = 45
  dimension "d141" = 275
  measures "d139" diameter of A48
extrude "Extrude11" cut sketch "To pass cables" against normal through all contours A48
mirror "Mirror11" about plane through (0, 0, 0) normal (1, 0, 0) of "Extrude11"
sketch "XZ bar" plane through (0, 8, 0) normal (0, 1, 0) x (-1, 0, 0)
  circle A0 centre (275, 101.5) radius 10
  circle A1 centre (-275, 101.5) radius 10
  circle A2 centre (133, 100) radius 1.5
  circle A3 centre (133, 60) radius 1.5
  circle A4 centre (133, 20) radius 1.5
  circle A5 centre (133, -20) radius 1.5
  circle A6 centre (133, -60) radius 1.5
  circle A7 centre (133, -100) radius 1.5
  circle A8 centre (133, -140) radius 1.5
  circle A9 centre (133, -180) radius 1.5
  circle A10 centre (133, -220) radius 1.5
  circle A11 centre (-133, 100) radius 1.5
  circle A12 centre (-133, 60) radius 1.5
  circle A13 centre (-133, 20) radius 1.5
  circle A14 centre (-133, -20) radius 1.5
  circle A15 centre (-133, -60) radius 1.5
  circle A16 centre (-133, -100) radius 1.5
  circle A17 centre (-133, -140) radius 1.5
  circle A18 centre (-133, -180) radius 1.5
  circle A19 centre (-133, -220) radius 1.5
  circle A20 centre (149, 260) radius 2.5
  circle A21 centre (117, 260) radius 2.5
  circle A22 centre (-149, 260) radius 2.5
  circle A23 centre (-117, 260) radius 2.5
  circle A24 centre (149, -260) radius 2.5
  circle A25 centre (117, -260) radius 2.5
  circle A26 centre (-149, -260) radius 2.5
  circle A27 centre (-117, -260) radius 2.5
  circle A28 centre (-242, -225.25) radius 2
  circle A29 centre (-242, -125.75) radius 2
  circle A30 centre (-242, -26.25) radius 2
  circle A31 centre (242, -225.25) radius 2
  circle A32 centre (242, -125.75) radius 2
  circle A33 centre (242, -26.25) radius 2
  circle A34 centre (-242, 133.875) radius 2
  circle A35 centre (-242, 214.625) radius 2
  circle A36 centre (-242, 58.5) radius 2
  circle A37 centre (-242, 290) radius 2
  line L0 (-246, 118.5) -> (-238, 118.5)
  line L1 (-238, 118.5) -> (-238, 68.5)
  line L2 (-238, 68.5) -> (-246, 68.5)
  line L3 (-246, 68.5) -> (-246, 118.5)
  line L4 (-238, 199.25) -> (-238, 149.25)
  line L5 (-238, 149.25) -> (-246, 149.25)
  line L6 (-246, 149.25) -> (-246, 199.25)
  line L7 (-246, 199.25) -> (-238, 199.25)
  line L8 (-238, 280) -> (-238, 230)
  line L9 (-238, 230) -> (-246, 230)
  line L10 (-246, 230) -> (-246, 280)
  line L11 (-246, 280) -> (-238, 280)
  circle A38 centre (242, 133.875) radius 2
  circle A39 centre (242, 214.625) radius 2
  circle A40 centre (242, 58.5) radius 2
  circle A41 centre (242, 290) radius 2
  line L12 (246, 68.5) -> (238, 68.5)
  line L13 (238, 68.5) -> (238, 118.5)
  line L14 (238, 118.5) -> (246, 118.5)
  line L15 (246, 118.5) -> (246, 68.5)
  line L16 (246, 199.25) -> (246, 149.25)
  line L17 (246, 149.25) -> (238, 149.25)
  line L18 (238, 149.25) -> (238, 199.25)
  line L19 (238, 199.25) -> (246, 199.25)
  line L20 (246, 280) -> (246, 230)
  line L21 (246, 230) -> (238, 230)
  line L22 (238, 230) -> (238, 280)
  line L23 (238, 280) -> (246, 280)
  circle A42 centre (291.5, 296) radius 2
  circle A43 centre (254.5, 296) radius 2
  circle A44 centre (-291.5, 52.5) radius 2
  line L24 (-260.5, 48.5) -> (-285.5, 48.5)
  line L25 (-285.5, 48.5) -> (-285.5, 56.5)
  line L26 (-285.5, 56.5) -> (-260.5, 56.5)
  line L27 (-260.5, 56.5) -> (-260.5, 48.5)
  circle A45 centre (-254.5, 52.5) radius 2
  circle A46 centre (291.5, 52.5) radius 2
  line L28 (260.5, 56.5) -> (285.5, 56.5)
  line L29 (285.5, 56.5) -> (285.5, 48.5)
  line L30 (285.5, 48.5) -> (260.5, 48.5)
  line L31 (260.5, 48.5) -> (260.5, 56.5)
  circle A47 centre (254.5, 52.5) radius 2
  line L32 (-260.5, 300) -> (-260.5, 292)
  line L33 (-260.5, 292) -> (-285.5, 292)
  line L34 (-285.5, 292) -> (-285.5, 300)
  line L35 (-285.5, 300) -> (-300, 300)
  line L36 (-300, 300) -> (-300, -36.5)
  line L37 (-300, -36.5) -> (-246, -36.5)
  line L38 (-246, -36.5) -> (-246, -51)
  line L39 (-238, -300) -> (238, -300)
  line L40 (246, -250) -> (246, -200.5)
  line L41 (246, -36.5) -> (300, -36.5)
  line L42 (300, -36.5) -> (300, 300)
  line L43 (300, 300) -> (285.5, 300)
  line L44 (285.5, 300) -> (285.5, 292)
  line L45 (285.5, 292) -> (260.5, 292)
  line L46 (260.5, 292) -> (260.5, 300)
  line L47 (260.5, 300) -> (-260.5, 300)
  circle A48 centre (-254.5, 296) radius 2
  circle A49 centre (-291.5, 296) radius 2
  circle A50 centre (-275, 28.5) radius 4
  circle A51 centre (133, 140) radius 1.5
  circle A52 centre (-133, 140) radius 1.5
  circle A53 centre (133, 180) radius 1.5
  circle A54 centre (-133, 180) radius 1.5
  circle A55 centre (16, -292.5) radius 2
  circle A56 centre (-16, -292.5) radius 2
  circle A57 centre (133, 220) radius 1.5
  circle A58 centre (-133, 220) radius 1.5
  line L48 (246, -1.5) -> (238, -1.5)
  line L49 (238, -1.5) -> (238, 48.5)
  line L50 (238, 48.5) -> (246, 48.5)
  line L51 (246, 48.5) -> (246, -1.5)
  line L52 (-246, 48.5) -> (-238, 48.5)
  line L53 (-238, 48.5) -> (-238, -1.5)
  line L54 (-238, -1.5) -> (-246, -1.5)
  line L55 (-246, -1.5) -> (-246, 48.5)
  line L56 (-246, -250) -> (-238, -250)
  line L57 (-238, -250) -> (-238, -300)
  line L58 (238, -300) -> (238, -250)
  line L59 (238, -250) -> (246, -250)
  line L60 (246, -200.5) -> (238, -200.5)
  line L61 (238, -200.5) -> (238, -150.5)
  line L62 (238, -150.5) -> (246, -150.5)
  line L63 (246, -150.5) -> (246, -101)
  line L64 (246, -101) -> (238, -101)
  line L65 (238, -101) -> (238, -51)
  line L66 (238, -51) -> (246, -51)
  line L67 (246, -51) -> (246, -36.5)
  line L68 (-246, -51) -> (-238, -51)
  line L69 (-238, -51) -> (-238, -101)
  line L70 (-238, -101) -> (-246, -101)
  line L71 (-246, -101) -> (-246, -150.5)
  line L72 (-246, -150.5) -> (-238, -150.5)
  line L73 (-238, -150.5) -> (-238, -200.5)
  line L74 (-238, -200.5) -> (-246, -200.5)
  line L75 (-246, -200.5) -> (-246, -250)
  dimension "d144" = 8
  dimension "d145" = 20
  dimension "d146" = 275
  measures "d144" diameter of A50
extrude "Extrude12" cut sketch "XZ bar" against normal through all contours A50
mirror "Mirror12" about plane through (0, 0, 0) normal (1, 0, 0) of "Extrude12"
sketch "XZ motor holes" plane through (0, 8, 0) normal (0, 1, 0) x (-1, 0, 0)
  circle A0 centre (275, 28.5) radius 4
  circle A1 centre (-275, 28.5) radius 4
  circle A2 centre (275, 101.5) radius 10
  circle A3 centre (-275, 101.5) radius 10
  circle A4 centre (133, 100) radius 1.5
  circle A5 centre (133, 60) radius 1.5
  circle A6 centre (133, 20) radius 1.5
  circle A7 centre (133, -20) radius 1.5
  circle A8 centre (133, -60) radius 1.5
  circle A9 centre (133, -100) radius 1.5
  circle A10 centre (133, -140) radius 1.5
  circle A11 centre (133, -180) radius 1.5
  circle A12 centre (133, -220) radius 1.5
  circle A13 centre (-133, 100) radius 1.5
  circle A14 centre (-133, 60) radius 1.5
  circle A15 centre (-133, 20) radius 1.5
  circle A16 centre (-133, -20) radius 1.5
  circle A17 centre (-133, -60) radius 1.5
  circle A18 centre (-133, -100) radius 1.5
  circle A19 centre (-133, -140) radius 1.5
  circle A20 centre (-133, -180) radius 1.5
  circle A21 centre (-133, -220) radius 1.5
  circle A22 centre (149, 260) radius 2.5
  circle A23 centre (117, 260) radius 2.5
  circle A24 centre (-149, 260) radius 2.5
  circle A25 centre (-117, 260) radius 2.5
  circle A26 centre (149, -260) radius 2.5
  circle A27 centre (117, -260) radius 2.5
  circle A28 centre (-149, -260) radius 2.5
  circle A29 centre (-117, -260) radius 2.5
  circle A30 centre (-242, -225.25) radius 2
  circle A31 centre (-242, -125.75) radius 2
  circle A32 centre (-242, -26.25) radius 2
  circle A33 centre (242, -225.25) radius 2
  circle A34 centre (242, -125.75) radius 2
  circle A35 centre (242, -26.25) radius 2
  circle A36 centre (-242, 133.875) radius 2
  circle A37 centre (-242, 214.625) radius 2
  circle A38 centre (-242, 58.5) radius 2
  circle A39 centre (-242, 290) radius 2
  line L0 (-246, 118.5) -> (-238, 118.5)
  line L1 (-238, 118.5) -> (-238, 68.5)
  line L2 (-238, 68.5) -> (-246, 68.5)
  line L3 (-246, 68.5) -> (-246, 118.5)
  line L4 (-238, 199.25) -> (-238, 149.25)
  line L5 (-238, 149.25) -> (-246, 149.25)
  line L6 (-246, 149.25) -> (-246, 199.25)
  line L7 (-246, 199.25) -> (-238, 199.25)
  line L8 (-238, 280) -> (-238, 230)
  line L9 (-238, 230) -> (-246, 230)
  line L10 (-246, 230) -> (-246, 280)
  line L11 (-246, 280) -> (-238, 280)
  circle A40 centre (242, 133.875) radius 2
  circle A41 centre (242, 214.625) radius 2
  circle A42 centre (242, 58.5) radius 2
  circle A43 centre (242, 290) radius 2
  line L12 (246, 68.5) -> (238, 68.5)
  line L13 (238, 68.5) -> (238, 118.5)
  line L14 (238, 118.5) -> (246, 118.5)
  line L15 (246, 118.5) -> (246, 68.5)
  line L16 (246, 199.25) -> (246, 149.25)
  line L17 (246, 149.25) -> (238, 149.25)
  line L18 (238, 149.25) -> (238, 199.25)
  line L19 (238, 199.25) -> (246, 199.25)
  line L20 (246, 280) -> (246, 230)
  line L21 (246, 230) -> (238, 230)
  line L22 (238, 230) -> (238, 280)
  line L23 (238, 280) -> (246, 280)
  circle A44 centre (291.5, 296) radius 2
  circle A45 centre (254.5, 296) radius 2
  circle A46 centre (-291.5, 52.5) radius 2
  line L24 (-260.5, 48.5) -> (-285.5, 48.5)
  line L25 (-285.5, 48.5) -> (-285.5, 56.5)
  line L26 (-285.5, 56.5) -> (-260.5, 56.5)
  line L27 (-260.5, 56.5) -> (-260.5, 48.5)
  circle A47 centre (-254.5, 52.5) radius 2
  circle A48 centre (291.5, 52.5) radius 2
  line L28 (260.5, 56.5) -> (285.5, 56.5)
  line L29 (285.5, 56.5) -> (285.5, 48.5)
  line L30 (285.5, 48.5) -> (260.5, 48.5)
  line L31 (260.5, 48.5) -> (260.5, 56.5)
  circle A49 centre (254.5, 52.5) radius 2
  line L32 (-260.5, 300) -> (-260.5, 292)
  line L33 (-260.5, 292) -> (-285.5, 292)
  line L34 (-285.5, 292) -> (-285.5, 300)
  line L35 (-285.5, 300) -> (-300, 300)
  line L36 (-300, 300) -> (-300, -36.5)
  line L37 (-300, -36.5) -> (-246, -36.5)
  line L38 (-246, -36.5) -> (-246, -51)
  line L39 (-238, -300) -> (238, -300)
  line L40 (246, -250) -> (246, -200.5)
  line L41 (246, -36.5) -> (300, -36.5)
  line L42 (300, -36.5) -> (300, 300)
  line L43 (300, 300) -> (285.5, 300)
  line L44 (285.5, 300) -> (285.5, 292)
  line L45 (285.5, 292) -> (260.5, 292)
  line L46 (260.5, 292) -> (260.5, 300)
  line L47 (260.5, 300) -> (-260.5, 300)
  circle A50 centre (-254.5, 296) radius 2
  circle A51 centre (-291.5, 296) radius 2
  line L48 (-290.5, 0.15) -> (-259.5, 0.15) construction
  line L49 (-259.5, 0.15) -> (-259.5, -30.85) construction
  line L50 (-259.5, -30.85) -> (-290.5, -30.85) construction
  line L51 (-290.5, -30.85) -> (-290.5, 0.15) construction
  circle A52 centre (-275, -15.35) radius 14
  circle A53 centre (-290.5, 0.15) radius 1.5
  circle A54 centre (-259.5, 0.15) radius 1.5
  circle A55 centre (-259.5, -30.85) radius 1.5
  circle A56 centre (-290.5, -30.85) radius 1.5
  circle A57 centre (133, 140) radius 1.5
  circle A58 centre (-133, 140) radius 1.5
  circle A59 centre (133, 180) radius 1.5
  circle A60 centre (-133, 180) radius 1.5
  circle A61 centre (16, -292.5) radius 2
  circle A62 centre (-16, -292.5) radius 2
  circle A63 centre (133, 220) radius 1.5
  circle A64 centre (-133, 220) radius 1.5
  line L52 (246, -1.5) -> (238, -1.5)
  line L53 (238, -1.5) -> (238, 48.5)
  line L54 (238, 48.5) -> (246, 48.5)
  line L55 (246, 48.5) -> (246, -1.5)
  line L56 (-246, 48.5) -> (-238, 48.5)
  line L57 (-238, 48.5) -> (-238, -1.5)
  line L58 (-238, -1.5) -> (-246, -1.5)
  line L59 (-246, -1.5) -> (-246, 48.5)
  line L60 (-246, -250) -> (-238, -250)
  line L61 (-238, -250) -> (-238, -300)
  line L62 (238, -300) -> (238, -250)
  line L63 (238, -250) -> (246, -250)
  line L64 (246, -200.5) -> (238, -200.5)
  line L65 (238, -200.5) -> (238, -150.5)
  line L66 (238, -150.5) -> (246, -150.5)
  line L67 (246, -150.5) -> (246, -101)
  line L68 (246, -101) -> (238, -101)
  line L69 (238, -101) -> (238, -51)
  line L70 (238, -51) -> (246, -51)
  line L71 (246, -51) -> (246, -36.5)
  line L72 (-246, -51) -> (-238, -51)
  line L73 (-238, -51) -> (-238, -101)
  line L74 (-238, -101) -> (-246, -101)
  line L75 (-246, -101) -> (-246, -150.5)
  line L76 (-246, -150.5) -> (-238, -150.5)
  line L77 (-238, -150.5) -> (-238, -200.5)
  line L78 (-238, -200.5) -> (-246, -200.5)
  line L79 (-246, -200.5) -> (-246, -250)
  dimension "d149" = 31
  dimension "d150" = 31
  dimension "d151" = 28
  dimension "d152" = 3
  dimension "d153" = 3
  dimension "d154" = 3
  dimension "d155" = 3
  dimension "d156" = 284.65
  dimension "d157" = 15.35
  measures "d151" diameter of A52
  measures "d152" diameter of A53
  measures "d153" diameter of A54
  measures "d154" diameter of A55
  measures "d155" diameter of A56
  measures "d157" distance of origin
extrude "Extrude13" cut sketch "XZ motor holes" against normal through all contours A52 | A53 | A54 | A55 | A56
mirror "Mirror13" about plane through (0, 0, 0) normal (1, 0, 0) of "Extrude13"